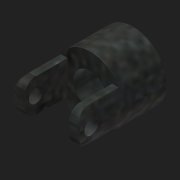
# Autodesk Inventor part: P1
Saved by Autodesk Inventor 2017 SP1 (Build 210196100, 196)
## iProperties
Created: 2018-03-20
Part Number: P1
Material: Steel
Document SubType Name: Modeling
Designer: Zach
Density: 7.85 g/cm^3
Appearance: Smooth - Black
Author: Zach
Autodesk Inventor part; units mm, degrees
ref_plane "YZ Plane" through (0, 0, 0) normal (1, 0, 0) x (0, 1, 0)
ref_plane "XZ Plane" through (0, 0, 0) normal (0, 1, 0) x (-1, 0, 0)
ref_plane "XY Plane" through (0, 0, 0) normal (0, 0, 1) x (1, 0, 0)
sketch "Sketch1" plane through (0, 0, 0) normal (0, 0, 1) x (1, 0, 0)
  circle A0 centre (0, 0) radius 6
  circle A1 centre (0, 0) radius 3
  dimension "d0" = 12
  dimension "d1" = 6
  constraints: 2 centre point, 2 coincident
  measures "d0" diameter of A0
  measures "d1" diameter of A1
extrude "Extrusion1" add sketch "Sketch1" along normal blind 15.5
sketch "Sketch2" plane through (0, 0, 15.5) normal (0, 0, 1) x (1, 0, 0)
  line L0 (-4, 6) -> (4, 6)
  line L1 (4, 6) -> (4, -6)
  line L2 (4, -6) -> (-4, -6)
  line L3 (-4, -6) -> (-4, 6)
  circle A0 centre (0, 0) radius 6 construction
  point P0 (0, 6)
  point P1 (4, 0)
  point P2 (0, -6)
  dimension "d4" = 8
  constraints: 8 end point, 3 midpoint, 2 parallel, 2 vertical alignment, 1 horizontal, 1 horizontal alignment, 1 perpendicular, 1 other
  measures "d4" distance of L0.start L0.end
extrude "Extrusion2" cut sketch "Sketch2" against normal blind 7.75
sketch "Sketch3" plane through (-4, -4.4721, 15.5) normal (1, 0, 0) x (0, 0, -1)
  arc A0 (2, 8.9443) -> (0, 6.9443) centre (2, 6.9443) ccw
  line L0 (0, 0) -> (7.75, 0) projected
  line L1 (7.75, 0) -> (7.75, 0) projected
  line L2 (7.75, 0) -> (0, 0) projected
  line L3 (0, 8.9443) -> (0, 0) projected
  line L4 (0, 8.9443) -> (7.75, 8.9443) projected
  line L5 (7.75, 8.9443) -> (7.75, 8.9443) projected
  line L6 (7.75, 8.9443) -> (0, 8.9443) projected
  line L7 (0, 0) -> (0, 8.9443) projected
  line L8 (15.5, -1.5279) -> (15.5, 10.4721) projected
  line L9 (0, 8.9443) -> (0, 0) projected
  arc A1 (0, 2) -> (2, 0) centre (2, 2) ccw
  line L10 (0, 2) -> (0, 0)
  line L11 (2, 0) -> (0, 0)
  line L12 (0, 6.9443) -> (0, 8.9443)
  line L13 (2, 8.9443) -> (0, 8.9443)
  point P0 (15.5, 4.4721)
  dimension "d7" = 2
  dimension "d8" = 2
  constraints: 8 end point, 7 tangent, 6 point on line, 4 collinear, 4 point on circle, 2 centre point
  measures "d7" radius of A0
  measures "d8" radius of A1
extrude "Extrusion3" cut sketch "Sketch3" along normal through all both and the other way through all
sketch "Sketch4" plane through (-4, -4.4721, 7.75) normal (1, 0, 0) x (0, 0, -1)
  circle A0 centre (-5.75, 4.4721) radius 1.25
  line L0 (-7.75, 6.9443) -> (-7.75, 2) projected
  point P0 (7.75, 4.4721)
  point P1 (-7.75, 4.4721)
  dimension "d11" = 2.5
  dimension "d12" = 2
  constraints: 1 centre point, 1 horizontal alignment, 1 midpoint
  measures "d11" diameter of A0
  measures "d12" distance from line of L0 A0.centre
extrude "Extrusion4" cut sketch "Sketch4" along normal through all both and the other way through all
sketch "Sketch5" plane through (0, 0, 7.75) normal (0, 0, 1) x (1, 0, 0)
  line L0 (-6, 3) -> (6, 3)
  line L1 (6, 3) -> (6, -3)
  line L2 (6, -3) -> (-6, -3)
  line L3 (-6, -3) -> (-6, 3)
  arc A0 (-5.467, 2.4721) -> (-5.467, -2.4721) centre (0, 0) ccw projected
  arc A1 (5.467, -2.4721) -> (5.467, 2.4721) centre (0, 0) ccw projected
  line L4 (-12.5137, 9.699) -> (15.0071, 9.699)
  line L5 (15.0071, 9.699) -> (15.0071, -9.2746)
  line L6 (15.0071, -9.2746) -> (-12.5137, -9.2746)
  line L7 (-12.5137, -9.2746) -> (-12.5137, 9.699)
  point P0 (0, 3)
  point P1 (-6, 0)
  dimension "d15" = 6
  constraints: 16 end point, 4 parallel, 2 horizontal, 2 midpoint, 2 perpendicular, 1 horizontal alignment, 1 point on circle, 1 vertical alignment
  measures "d15" distance of L0.end L1.end
extrude "Extrusion5" cut sketch "Sketch5" along normal through all
fillet "Fillet1" radius 2 4 edges at (-4.5981, 3, 15.4291) (-4.5981, -3, 15.4291) (4.5981, 3, 15.4291) (4.5981, -3, 15.4291)
body "Solid1"
